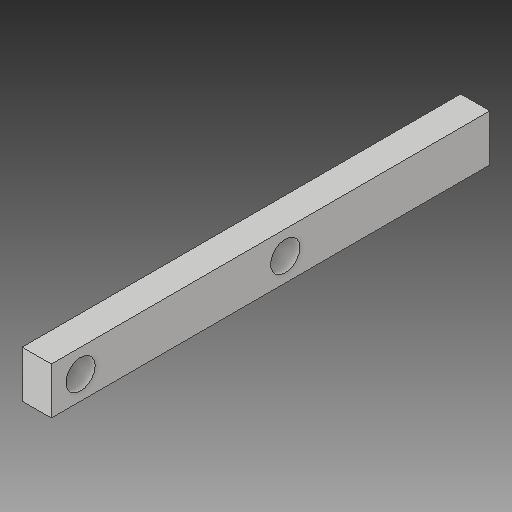
# Autodesk Inventor part: Haste
Saved by Autodesk Inventor 2019 (Build 230136000, 136)
## iProperties
Created: 2020-04-04
Part Number: Haste
Material: Generic
Document SubType Name: Modeling
Designer: Hermann
Density: 1 g/cm^3
Appearance: Default
Author: Hermann
Autodesk Inventor part; units mm, degrees
ref_plane "YZ Plane" through (0, 0, 0) normal (1, 0, 0) x (0, 1, 0)
ref_plane "XZ Plane" through (0, 0, 0) normal (0, 1, 0) x (-1, 0, 0)
ref_plane "XY Plane" through (0, 0, 0) normal (0, 0, 1) x (1, 0, 0)
sketch "Sketch1" plane through (0, 0, 0) normal (1, 0, 0) x (0, 1, 0)
  line L0 (8, 10) -> (-8, 10)
  line L1 (-8, 10) -> (-8, -140)
  line L2 (-8, -140) -> (8, -140)
  line L3 (8, -140) -> (8, 10)
  point P0 (0, 0)
  dimension "d0" = 16
  dimension "d1" = 8
  dimension "d2" = 10
  dimension "d3" = 150
  constraints: 8 end point, 2 parallel, 1 horizontal, 1 perpendicular
  measures "d0" distance between parallel lines of L1 L3
  measures "d1" distance from line of L3 point (0, 0)
  measures "d2" distance from line of point (0, 0) L0
  measures "d3" distance between parallel lines of L0 L2
extrude "Extrusion1" add sketch "Sketch1" along normal blind 10
sketch "Sketch2" plane through (10, 0, 0) normal (1, 0, 0) x (0, 0, -1)
  point P0 (0, 0)
  point P1 (0, 0)
  constraints: 1 coincident
hole "Hole1" at (10, 0, 0) direction (-1, 0, 0) diameter 10 depth 22 tip angle 118
sketch "Sketch3" plane through (10, 0, 0) normal (1, 0, 0) x (0, 0, -1)
  point P0 (0, 0)
  point P1 (70, 0)
  dimension "d20" = 0
  dimension "d21" = 70
  measures "d20" vertical distance of point (0, 0) point (70, 0)
  measures "d21" distance of point (0, 0) point (70, 0)
hole "Hole2" at (10, 0, -70) direction (-1, 0, 0) diameter 10 depth 22 tip angle 118
body "Solid1"
